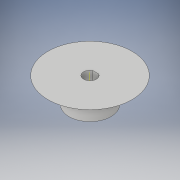
# Autodesk Inventor part: spool
Saved by Autodesk Inventor 2019 (Build 230136000, 136)
## iProperties
Created: 2019-01-26
Part Number: spool
Material: Generic
Document SubType Name: Modeling
Designer: User
Density: 1 g/cm^3
Appearance: Default
Author: User
Autodesk Inventor part; units mm, degrees
ref_plane "YZ Plane" through (0, 0, 0) normal (1, 0, 0) x (0, 1, 0)
ref_plane "XZ Plane" through (0, 0, 0) normal (0, 1, 0) x (-1, 0, 0)
ref_plane "XY Plane" through (0, 0, 0) normal (0, 0, 1) x (1, 0, 0)
sketch "Sketch4" plane through (0, 0, 0) normal (1, 0, 0) x (0, 1, 0)
  line L0 (0, 0) -> (0, -9.525)
  line L1 (0, 0) -> (11.43, 0)
  line L2 (11.43, 0) -> (11.43, -19.05)
  arc A0 (11.43, -19.05) -> (0, -9.525) centre (-2.6269, -24.2978) ccw
  dimension "d18" = 9.525
  dimension "d19" = 11.43
  dimension "d20" = 19.05
  constraints: 6 end point, 2 point on circle, 1 centre point, 1 horizontal, 1 perpendicular, 1 vertical
  measures "d18" distance of L0.start L0.end
  measures "d19" distance of L0.start L1.end
  measures "d20" distance of L1.end L2.end
revolve "Revolution1" add sketch "Sketch4" angle 360 about axis through (0, 0, 0) along (0, 1, 0)
sketch "Sketch5" plane through (0, 11.43, 0) normal (0, 1, 0) x (1, 0, 0)
  circle A0 centre (0, 0) radius 2.921
  line L0 (-1.3968, 2.5654) -> (1.3968, 2.5654)
  dimension "d22" = 5.842
  dimension "d23" = 2.5654
  constraints: 2 end point, 2 point on circle, 1 centre point, 1 coincident, 1 horizontal
  measures "d22" diameter of A0
  measures "d23" distance from line of point (0, 0) L0
extrude "Extrusion1" cut sketch "Sketch5" against normal through all contours A0 L0 picked at (-0.1728, -0.6264)
body "Solid2"
